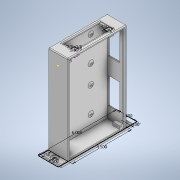
# Autodesk Inventor part: Video-UI Module for RoadBot Rail-r3
Saved by Autodesk Inventor 2020 (Build 240168000, 168)
## iProperties
Created: 2022-03-30
Part Number: Video-UI Module for RoadBot Rail-r3
Material: Generic
Document SubType Name: Modeling
Designer: Beaucage
Density: 1 g/cm^3
Appearance: Default
Author: Beaucage
Autodesk Inventor part; units mm, degrees
ref_plane "YZ Plane" through (0, 0, 0) normal (1, 0, 0) x (0, 1, 0)
ref_plane "XZ Plane" through (0, 0, 0) normal (0, 1, 0) x (-1, 0, 0)
ref_plane "XY Plane" through (0, 0, 0) normal (0, 0, 1) x (1, 0, 0)
sketch "Sketch1" plane through (0, 0, 0) normal (0, 1, 0) x (-1, 0, 0)
  line L0 (0, 0) -> (38.1, 0)
  line L1 (38.1, 0) -> (38.1, -152.4)
  line L2 (38.1, -152.4) -> (0, -152.4)
  line L3 (0, -152.4) -> (0, 0)
  line L4 (38.1, 0) -> (38.1, -19.05)
  line L5 (38.1, -19.05) -> (0, -19.05)
  line L6 (0, -19.05) -> (0, -133.35)
  line L7 (0, -133.35) -> (38.1, -133.35)
  line L8 (38.1, -133.35) -> (38.1, -19.05)
  line L9 (19.05, -152.4) -> (19.05, -139.7)
  line L10 (19.05, 0) -> (19.05, -12.7)
  line L11 (19.05, 0) -> (31.75, 0) construction
  point P0 (38.1, -133.35)
  point P1 (0, -19.05)
  point P2 (38.1, -9.525)
  dimension "d0" = 38.1
  dimension "d1" = 152.4
  dimension "d2" = 19.05
  dimension "d3" = 114.3
  dimension "d8" = 12.7
  dimension "d41" = 12.7
  constraints: 24 end point, 4 parallel, 4 perpendicular, 3 horizontal, 2 midpoint, 2 point on line, 1 vertical
  measures "d0" distance of L1.end L2.end
  measures "d1" distance of L0.end L1.end
  measures "d2" distance of L0.end L4.end
  measures "d3" distance of L6.end L5.end
  measures "d8" distance of L9.start L9.end
  measures "d41" distance of L10.start L10.end
extrude "Extrusion1" add sketch "Sketch1" against normal blind 4.7625
extrude "Extrusion2" add sketch "Sketch1" along normal blind 171.45 contours L5 L1 L7 L3
hole "Hole1" at (-19.05, 0, -12.7) at (-19.05, 0, -139.7) direction (0, -1, 0) diameter 6.7564 end through all counterbore diameter 12.8778 counterbore depth 1.5875 clearance for "Flat Head Machine Screw (82)" size "1/4" standard "Ansi Unified Screw Threads"
sketch "Sketch7" plane through (-38.1, 0, 0) normal (0, 0, 1) x (1, 0, 0)
  line L0 (38.1, -4.7625) -> (0, -4.7625) projected
  line L1 (-38.1, 0) -> (38.1, 0)
  line L2 (38.1, 0) -> (38.1, -4.7625)
  line L3 (38.1, -4.7625) -> (-38.1, -4.7625)
  line L4 (-38.1, -4.7625) -> (-38.1, 0)
  line L5 (38.1, 0) -> (38.1, 171.45) projected
  line L6 (38.1, 0) -> (0, 0)
  line L7 (0, 0) -> (0, -4.7625)
  line L8 (0, -4.7625) -> (38.1, -4.7625)
  line L9 (38.1, -4.7625) -> (38.1, 0)
  constraints: 16 end point, 4 parallel, 2 horizontal, 2 perpendicular
extrude "Extrusion7" cut sketch "Sketch7" against normal blind 6.35 contours L0 L7 L1 L2
sketch "Sketch8" plane through (0, 0, -152.4) normal (0, 0, -1) x (-1, 0, 0)
  line L0 (0, -4.7625) -> (38.1, -4.7625) projected
  line L1 (0, 0) -> (0, -4.7625) projected
  line L2 (38.1, -4.7625) -> (0, -4.7625)
  line L3 (0, -4.7625) -> (0, 0)
  line L4 (0, 0) -> (38.1, 0)
  line L5 (38.1, 0) -> (38.1, -4.7625)
  point P0 (15.6718, -4.7625)
  constraints: 8 end point, 2 parallel, 1 horizontal, 1 perpendicular
extrude "Extrusion8" cut sketch "Sketch8" against normal blind 6.35
sketch "Sketch2" plane through (0, -4.7625, 0) normal (1, 0, 0) x (0, 0, -1)
  line L0 (133.35, 4.7625) -> (133.35, 176.2125) projected
  line L1 (133.35, 176.2125) -> (128.5875, 176.2125)
  line L2 (19.05, 176.2125) -> (133.35, 176.2125) projected
  line L3 (128.5875, 176.2125) -> (128.5875, 171.45)
  line L4 (19.05, 4.8538) -> (23.8125, 4.8538)
  line L5 (23.8125, 4.8538) -> (128.5875, 4.8538)
  line L6 (128.5875, -1.5875) -> (128.5875, 171.45)
  line L7 (128.5875, 171.45) -> (23.8125, 171.45)
  line L8 (23.8125, 171.45) -> (23.8125, -1.5875)
  point P0 (0, 4.7625)
  dimension "d16" = 4.7625
  dimension "d17" = 4.7625
  dimension "d18" = 4.7625
  constraints: 14 end point, 2 horizontal, 2 parallel, 1 perpendicular, 1 point on line, 1 vertical
  measures "d16" distance of L0.end L1.end
  measures "d17" distance of L1.end L3.end
  measures "d18" distance of L4.start L4.end
extrude "Extrusion3" cut sketch "Sketch2" against normal blind 33.3375
sketch "Sketch3" plane through (0, -4.7625, 0) normal (1, 0, 0) x (0, 0, -1)
  line L0 (19.05, 176.2125) -> (133.35, 176.2125) projected
  line L1 (133.35, 176.2125) -> (130.175, 176.2125)
  line L2 (130.175, 176.2125) -> (130.175, 173.0375)
  line L3 (152.4, 0) -> (0, 0) projected
  line L4 (19.05, 0) -> (22.225, 0)
  line L5 (22.225, 0) -> (22.225, 3.175)
  line L6 (130.175, 173.0375) -> (22.225, 173.0375)
  line L7 (22.225, 173.0375) -> (22.225, 3.175)
  line L8 (22.225, 3.175) -> (130.175, 3.175)
  line L9 (130.175, 3.175) -> (130.175, 173.0375)
  point P0 (0, 4.7625)
  dimension "d21" = 3.175
  dimension "d22" = 3.175
  dimension "d23" = 3.175
  dimension "d24" = 3.175
  constraints: 16 end point, 3 perpendicular, 3 point on line, 2 parallel, 1 horizontal
  measures "d21" distance of L0.end L1.end
  measures "d22" distance of L1.end L2.end
  measures "d23" distance of L4.start L4.end
  measures "d24" distance of L4.end L5.end
extrude "Extrusion4" cut sketch "Sketch3" against normal blind 3.175
sketch "Sketch4" plane through (-33.3375, 0.0913, -23.8125) normal (0, 1, 0) x (1, 0, 0)
  line L0 (30.1625, 104.775) -> (0, 104.775) projected
  line L1 (30.1625, 104.775) -> (17.4625, 104.775)
  line L2 (17.4625, 104.775) -> (17.4625, 98.425)
  line L3 (17.4625, 98.425) -> (30.1625, 98.425)
  line L4 (30.1625, 98.425) -> (30.1625, 104.775)
  point P0 (33.3375, -23.8125)
  point P1 (55.5625, 104.775)
  point P2 (33.3375, 104.775)
  dimension "d27" = 12.7
  dimension "d28" = 6.35
  constraints: 8 end point, 2 parallel, 1 horizontal, 1 perpendicular
  measures "d27" distance of L3.end L2.end
  measures "d28" distance of L2.end L1.end
extrude "Extrusion5" add sketch "Sketch4" along normal blind 6.35
sketch "Sketch5" plane through (-33.3375, 166.6875, -128.5875) normal (0, -1, 0) x (1, 0, 0)
  line L0 (30.1625, 104.775) -> (17.4625, 104.775)
  line L1 (17.4625, 104.775) -> (17.4625, 98.425)
  line L2 (17.4625, 98.425) -> (30.1625, 98.425)
  line L3 (30.1625, 98.425) -> (30.1625, 104.775)
  point P0 (33.3375, 128.5875)
  dimension "d31" = 12.7
  dimension "d32" = 6.35
  constraints: 8 end point, 2 parallel, 1 horizontal, 1 perpendicular
  measures "d31" distance of L2.end L1.end
  measures "d32" distance of L1.end L0.end
extrude "Extrusion6" add sketch "Sketch5" along normal blind 6.35
sketch "Sketch6" plane through (-33.3375, -4.7625, 0) normal (1, 0, 0) x (0, 0, -1)
  line L0 (128.5875, 4.8538) -> (23.8125, 4.8538) projected
  line L1 (23.8125, 4.8538) -> (38.8125, 4.8538)
  line L2 (38.8125, 4.8538) -> (38.8125, 28.3538)
  line L3 (38.8125, 28.3538) -> (87.8125, 28.3538)
  line L4 (87.8125, 28.3538) -> (87.8125, 86.3538)
  line L5 (87.8125, 86.3538) -> (38.8125, 86.3538)
  line L6 (38.8125, 86.3538) -> (38.8125, 28.3538)
  circle A0 centre (38.8125, 28.3538) radius 2.5
  point P0 (0, 4.7625)
  dimension "d35" = 15
  dimension "d36" = 23.5
  dimension "d37" = 49
  dimension "d38" = 58
  dimension "d45" = 5
  constraints: 12 end point, 2 parallel, 1 centre point, 1 coincident, 1 horizontal, 1 perpendicular, 1 point on line, 1 vertical
  measures "d35" distance of L0.end L1.end
  measures "d36" distance of L1.end L2.end
  measures "d37" distance of L5.end L4.end
  measures "d38" distance of L4.end L3.end
  measures "d45" diameter of A0
extrude "Extrusion9" add sketch "Sketch6" along normal blind 2 contours A0 L6 L2 | L2 L3 A0 | L6 A0 L3
sketch "Sketch9" plane through (-31.3375, 23.5913, -38.8125) normal (1, 0, 0) x (0, 0, -1)
  point P0 (-38.8125, -23.5913)
  point P1 (0, 0)
  point P2 (0, 0)
  constraints: 1 coincident
hole "Hole2" at (-31.3375, 23.5913, -38.8125) direction (-1, 0, 0) diameter 2.05 depth 2 tip angle 118
thread "Thread1" size "M2.5x0.45" class "6H" standard "ANSI Metric M Profile" full length
pattern_linear "Rectangular Pattern1" count 2 spacing 58 along (0, 0, -1) count 2 spacing 49 along (0, 1, 0) of "Extrusion9", "Hole2"
sketch "Sketch12" plane through (-3.175, -4.7625, 0) normal (1, 0, 0) x (0, 0, -1)
  line L0 (22.225, 173.0375) -> (26.9875, 173.0375)
  line L1 (26.9875, 173.0375) -> (26.9875, 168.275)
  line L2 (26.9875, 168.275) -> (22.225, 168.275)
  line L3 (22.225, 168.275) -> (22.225, 173.0375)
  line L4 (122.2375, 4.8538) -> (122.2375, 11.2038) projected
  line L5 (122.2375, 11.2038) -> (125.4125, 11.2038)
  line L6 (125.4125, 11.2038) -> (125.4125, 8.0288)
  line L7 (125.4125, 8.0288) -> (122.2375, 8.0288)
  line L8 (122.2375, 8.0288) -> (122.2375, 11.2038)
  point P0 (0, 4.7625)
  dimension "d82" = 4.7625
  dimension "d83" = 4.7625
  dimension "d84" = 3.175
  dimension "d85" = 3.175
  constraints: 16 end point, 4 parallel, 2 horizontal, 2 perpendicular
  measures "d82" distance of L1.end L2.end
  measures "d83" distance of L0.end L1.end
  measures "d84" distance of L6.end L7.end
  measures "d85" distance of L5.end L6.end
hole "Hole4" at (-3.175, 163.5125, -26.9875) at (-3.175, 3.2663, -125.4125) direction (-1, 0, 0) diameter 2.2606 depth 5.6896 tip angle 118
fillet "Fillet1" radius 1.5875 16 edges at (-19.05, 171.45, -19.05) (0, 171.45, -76.2) (0, 85.725, -19.05) (0, 85.725, -133.35) (-19.05, 171.45, -133.35) (-38.1, 171.45, -76.2) (-38.1, 85.725, -133.35) (-8.9919, 0, -146.05) (-29.1081, 0, -146.05) (-29.1081, 0, -6.35) (-8.9919, 0, -6.35) (-38.1, 0, -139.7) (-38.1, 85.725, -19.05) (-38.1, 0, -12.7) (0, 0, -12.7) (0, 0, -139.7)
sketch "Sketch16" plane through (0, 171.45, 0) normal (0, 1, 0) x (1, 0, 0)
  line L0 (-38.1, 0) -> (-38.1, 146.05) projected
  line L1 (-38.1, 146.05) -> (-38.1, 76.2)
  line L2 (-38.1, 76.2) -> (-38.1, 114.3)
  line L3 (-38.1, 131.7625) -> (-38.1, 20.6375) projected
  line L4 (-38.1, 76.2) -> (-19.05, 76.2)
  line L5 (-38.1, 76.2) -> (-19.05, 76.2) construction
  line L6 (-6.35, 38.1) -> (-31.75, 38.1)
  line L7 (-31.75, 38.1) -> (-31.75, 114.3)
  line L8 (-31.75, 114.3) -> (-6.35, 114.3)
  line L9 (-6.35, 114.3) -> (-6.35, 38.1)
  line L10 (-6.35, 38.1) -> (-31.75, 114.3) construction
  line L11 (-31.75, 38.1) -> (-6.35, 114.3) construction
  point P0 (0, 0)
  point P1 (-38.1, 6.35)
  dimension "d128" = 69.85
  dimension "d130" = 19.05
  dimension "d131" = 0
  dimension "d132" = 25.4
  dimension "d133" = 76.2
  constraints: 20 end point, 3 horizontal, 2 midpoint, 2 parallel, 2 point on line, 1 collinear, 1 perpendicular
  measures "d128" distance of L0.end L1.end
  measures "d130" distance of L1.end L4.end
  measures "d131" distance between parallel lines of L4 L5
  measures "d132" distance of L7.end L8.end
  measures "d133" distance of L6.end L7.end
extrude "Extrusion11" cut sketch "Sketch16" against normal blind 1.5875
sketch "Sketch17" plane through (0, 169.8625, 0) normal (0, 1, 0) x (1, 0, 0)
  line L0 (-6.35, 38.1) -> (-31.75, 38.1) projected
  line L1 (-31.75, 38.1) -> (-31.75, 76.2)
  line L2 (-31.75, 38.1) -> (-31.75, 114.3) projected
  line L3 (-31.75, 76.2) -> (-19.05, 76.2)
  line L4 (-9.525, 41.275) -> (-28.575, 41.275)
  line L5 (-28.575, 41.275) -> (-28.575, 111.125)
  line L6 (-28.575, 111.125) -> (-9.525, 111.125)
  line L7 (-9.525, 111.125) -> (-9.525, 41.275)
  line L8 (-9.525, 41.275) -> (-28.575, 111.125) construction
  line L9 (-28.575, 41.275) -> (-9.525, 111.125) construction
  line L10 (-28.575, 41.275) -> (-31.75, 41.275)
  line L11 (-31.75, 41.275) -> (-31.75, 111.125)
  line L12 (-31.75, 111.125) -> (-28.575, 111.125)
  line L13 (-28.575, 111.125) -> (-28.575, 41.275)
  point P0 (0, 0)
  point P1 (-31.75, 41.275)
  point P2 (0, 38.1)
  dimension "d136" = 38.1
  dimension "d137" = 12.7
  dimension "d138" = 90
  dimension "d139" = 19.05
  dimension "d140" = 69.85
  constraints: 24 end point, 4 parallel, 3 midpoint, 3 perpendicular, 2 horizontal, 1 point on line
  measures "d136" distance of L0.end L1.end
  measures "d137" distance of L1.end L3.end
  measures "d138" angle of L1 L3
  measures "d139" distance of L5.end L6.end
  measures "d140" distance of L4.end L5.end
extrude "Extrusion12" cut sketch "Sketch17" against normal blind 3.175
sketch "Sketch18" plane through (0, 169.8625, 0) normal (0, 1, 0) x (1, 0, 0)
  line L0 (-6.35, 38.1) -> (-31.75, 38.1) projected
  line L1 (-6.35, 38.1) -> (-15.875, 38.1)
  line L2 (-15.875, 38.1) -> (-15.875, 47.625)
  line L3 (-15.875, 47.625) -> (-6.35, 47.625)
  line L4 (-6.35, 47.625) -> (-6.35, 38.1)
  line L5 (-6.35, 114.3) -> (-6.35, 38.1) projected
  line L6 (-6.35, 114.3) -> (-15.875, 114.3)
  line L7 (-15.875, 114.3) -> (-15.875, 104.775)
  line L8 (-15.875, 104.775) -> (-6.35, 104.775)
  line L9 (-6.35, 104.775) -> (-6.35, 114.3)
  line L10 (-6.35, 38.1) -> (-6.35, 42.8625)
  line L11 (-6.35, 42.8625) -> (-11.1125, 42.8625)
  line L12 (-6.35, 114.3) -> (-6.35, 109.5375)
  line L13 (-6.35, 109.5375) -> (-11.1125, 109.5375)
  point P0 (0, 0)
  point P1 (-6.35, 104.775)
  point P2 (-15.875, 38.1)
  point P3 (0, 38.1)
  dimension "d143" = 9.525
  dimension "d144" = 9.525
  dimension "d145" = 9.525
  dimension "d146" = 9.525
  dimension "d149" = 4.7625
  dimension "d150" = 4.7625
  dimension "d151" = 4.7625
  dimension "d152" = 4.7625
  constraints: 24 end point, 4 parallel, 4 perpendicular, 2 horizontal, 1 midpoint, 1 point on line
  measures "d143" distance of L2.end L3.end
  measures "d144" distance of L1.end L2.end
  measures "d145" distance of L8.end L7.end
  measures "d146" distance of L7.end L6.end
  measures "d149" distance of L0.start L10.end
  measures "d150" distance of L10.end L11.end
  measures "d151" distance of L5.start L12.end
  measures "d152" distance of L12.end L13.end
extrude "Extrusion13" add sketch "Sketch18" against normal blind 9.525
hole "Hole6" at (-11.1125, 169.8625, -42.8625) at (-11.1125, 169.8625, -109.5375) direction (0, -1, 0) diameter 2.2606 depth 6.5786 tip angle 118
fillet "Fillet2" radius 1.5875 2 edges at (-31.75, 171.45, -76.2) (-31.75, 166.6875, -76.2)
fillet "Fillet3" radius 3.175 4 edges at (-33.3375, 72.5913, -94.3125) (-33.3375, 72.5913, -36.3125) (-33.3375, 23.5913, -36.3125) (-33.3375, 23.5913, -94.3125)
pattern_linear "Rectangular Pattern3" count 2 spacing 85 along (0, 1, 0) of "Extrusion9", "Hole2", "Rectangular Pattern1"
fillet "Fillet4" radius 3.175 4 edges at (-33.3375, 157.5913, -36.3125) (-33.3375, 108.5913, -36.3125) (-33.3375, 108.5913, -94.3125) (-33.3375, 157.5913, -94.3125)
sketch "Sketch30" plane through (-1.5875, 169.8625, -133.35) normal (0, 0, -1) x (-1, 0, 0)
  line L0 (29.75, -147.2962) -> (29.75, -145.2462) projected
  line L1 (29.75, -98.2962) -> (29.75, -96.2462) projected
  line L2 (29.75, -62.2962) -> (29.75, -60.2462) projected
  line L3 (-1.5875, -1.5875) -> (-1.5875, -171.45) projected
  line L4 (29.75, -13.2962) -> (29.75, -11.2462) projected
  line L5 (29.75, -58.7712) -> (29.75, -63.7712) projected
  line L6 (29.75, -11.2462) -> (29.75, -63.7712)
  line L7 (29.75, -63.7712) -> (7.525, -63.7712)
  line L8 (7.525, -63.7712) -> (7.525, -11.2462)
  line L9 (7.525, -11.2462) -> (29.75, -11.2462)
  line L10 (29.75, -96.2462) -> (29.75, -147.2962)
  line L11 (29.75, -147.2962) -> (7.525, -147.2962)
  line L12 (7.525, -147.2962) -> (7.525, -96.2462)
  line L13 (7.525, -96.2462) -> (29.75, -96.2462)
  point P0 (-1.5875, -169.8625)
  dimension "d277" = 22.225
  dimension "d278" = 22.225
  constraints: 16 end point, 4 parallel, 2 perpendicular, 1 collinear, 1 vertical
  measures "d277" distance of L5.end L7.end
  measures "d278" distance of L0.start L11.end
extrude "Extrusion18" cut sketch "Sketch30" against normal up to surface (4.7625 mm away)
fillet "Fillet5" radius 3.175 8 edges at (-31.3375, 132.3538, -133.35) (-20.225, 158.6163, -133.35) (-9.1125, 132.3538, -133.35) (-20.225, 106.0913, -133.35) (-20.225, 73.6163, -133.35) (-9.1125, 48.0913, -133.35) (-31.3375, 48.0913, -133.35) (-20.225, 22.5663, -133.35)
equation "\"d206\" = 55deg"
equation "\"Sketch22_Pitch\" = 0.45"
equation "\"d224\" = 55deg"
equation "\"Sketch24_Pitch\" = 0.45"
equation "\"d244\" = 55deg"
equation "\"Sketch26_Pitch\" = 0.45"
equation "\"d262\" = 55deg"
equation "\"Sketch28_Pitch\" = 0.45"
body "Solid1"
